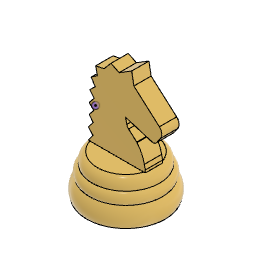
knight-piece (Autodesk Fusion 360 design; units mm, degrees)
Autodesk Fusion 360 part; units mm, degrees
sketch "Sketch1" plane through (0, 0, 0) normal (0, 1, 0) x (1, 0, 0)
  line L0 (0.63787, -5.613368) -> (1.322235, -4.705961)
  line L1 (1.781849, -13.501986) -> (2.054004, -12.134883)
  line L2 (4.431532, -15.195434) -> (3.230917, -13.790457)
  arc A0 (12.369222, -7.229903) -> (11.532634, -6.942255) centre (11.753991, -7.658845) ccw
  line L3 (0.654946, -7.413287) -> (1.44732, -6.605734)
  line L4 (7.495864, -6.835009) -> (8.909119, -5.586097)
  line L5 (11.532634, -6.942255) -> (6.964148, -8.353478)
  line L6 (12.782214, -7.990364) -> (12.77555, -7.981881)
  line L7 (0.992877, -11.410262) -> (1.682411, -10.30367)
  line L8 (12.846864, -9.85003) -> (8.411678, -13.769464)
  line L9 (2.054004, -12.134883) -> (0.992877, -11.410262)
  line L10 (8.94361, -5.555616) -> (9.013978, -5.467489)
  line L11 (0.773914, -9.412249) -> (1.492016, -8.460111)
  line L12 (13.044505, -8.198462) -> (12.369222, -7.229903)
  arc A1 (8.964814, -5.528278) -> (10.23694, -2.89688) centre (4.129914, -1.567691) ccw
  line L13 (5.849674, -14.499572) -> (4.431532, -15.195434)
  line L14 (1.322235, -4.705961) -> (0.495264, -3.671767)
  line L15 (1.304006, -2.784416) -> (0.492137, -1.671328)
  arc A2 (12.846864, -9.85003) -> (13.044505, -8.198462) centre (12.01912, -8.913365) ccw
  line L16 (3.230917, -13.790457) -> (1.781849, -13.501986)
  line L17 (6.964148, -8.353478) -> (7.181578, -7.368735)
  line L18 (10.404418, -1.671328) -> (10.404418, -2.127392)
  arc A3 (7.495864, -6.835009) -> (7.181578, -7.368735) centre (8.158059, -7.584341) ccw
  line L19 (1.492016, -8.460111) -> (0.654946, -7.413287)
  line L20 (8.411678, -13.769464) -> (8.035252, -15.843654)
  line L21 (0.495264, -3.671767) -> (1.304006, -2.784416)
  line L22 (1.44732, -6.605734) -> (0.63787, -5.613368)
  line L23 (8.035252, -15.843654) -> (5.849674, -14.499572)
  arc A4 (8.909119, -5.586097) -> (8.964814, -5.528278) centre (8.578022, -5.211431) ccw
  line L24 (10.23694, -2.89688) -> (10.404418, -2.127392)
  line L25 (1.682411, -10.30367) -> (0.773914, -9.412249)
  line L26 (0.492137, -1.671328) -> (10.404418, -1.671328)
  constraint perpendicular L1 L16
  constraint perpendicular L3 L25
  constraint parallel L0 L11
  constraint parallel L14 L19
  constraint parallel L4 L8
  constraint tangent A1 L24
  constraint tangent L10 A1
  constraint tangent L4 A3
  constraint tangent L17 A3
  constraint tangent L4 A4
  constraint tangent A1 A4
  constraint tangent L8 A2
  constraint tangent L12 A2
  constraint tangent A0 L5
  constraint tangent A0 L12
  constraint perpendicular L18 L26
extrude "Extrude3" add sketch "Sketch1" along normal blind 3 contours L0 L1 L2 A0 L3 L4 L5 L7 L8 L9 L10 L11 L12 A1 L13 L14 L15 A2 L16 L17 L18 A3 L19 L20 L21 L22 L23 A4 L24 L25 L26 picked at (9.407563, -10.657657)
sketch "Sketch4" plane through (0, 0, 0) normal (0, 1, 0) x (1, 0, 0)
sketch "Sketch5" plane through (0, 0, 0) normal (0, 1, 0) x (1, 0, 0)
scale "Scale1" factor 2.2 about (3.230917, 0, 13.790457) bodies 1
sketch "Sketch6" plane through (0, 0, 0) normal (0, -1, 0) x (1, 0, 0)
  arc A0 (24.820812, 1.488068) -> (24.386, 5.121516) centre (22.564965, 3.060854) ccw
  line L0 (24.386, 5.121516) -> (14.628591, 13.744271)
  line L1 (14.628591, 13.744271) -> (13.800454, 18.30749)
  line L2 (13.800454, 18.30749) -> (8.992182, 15.35051)
  line L3 (8.992182, 15.35051) -> (5.87227, 16.881406)
  line L4 (5.87227, 16.881406) -> (3.230917, 13.790457)
  line L5 (3.230917, 13.790457) -> (0.042969, 13.155821)
  line L6 (0.042969, 13.155821) -> (0.641708, 10.148194)
  line L7 (0.641708, 10.148194) -> (-1.692769, 8.554027)
  line L8 (-1.692769, 8.554027) -> (-0.175795, 6.119526)
  line L9 (-0.175795, 6.119526) -> (-2.174489, 4.158398)
  line L10 (-2.174489, 4.158398) -> (-0.594666, 2.063694)
  line L11 (-0.594666, 2.063694) -> (-2.43622, -0.239317)
  line L12 (-2.43622, -0.239317) -> (-0.692995, -2.015934)
  line L13 (-0.692995, -2.015934) -> (-2.473786, -4.199139)
  line L14 (-2.473786, -4.199139) -> (-0.968182, -6.195434)
  line L15 (-0.968182, -6.195434) -> (-2.787519, -8.47066)
  line L16 (-2.787519, -8.47066) -> (-1.008287, -10.422834)
  line L17 (-1.008287, -10.422834) -> (-2.794399, -12.871628)
  line L18 (-2.794399, -12.871628) -> (19.012619, -12.871628)
  line L19 (19.012619, -12.871628) -> (19.012619, -11.868286)
  line L20 (19.012619, -11.868286) -> (18.644167, -10.175413)
  arc A1 (18.644167, -10.175413) -> (15.845491, -4.386338) centre (5.208711, -13.099629) ccw
  arc A2 (15.845491, -4.386338) -> (15.722963, -4.259136) centre (14.994548, -5.083401) ccw
  line L21 (15.722963, -4.259136) -> (12.613801, -1.511528)
  arc A3 (11.922372, -0.337331) -> (12.613801, -1.511528) centre (14.070629, 0.137002) ccw
  line L22 (11.922372, -0.337331) -> (11.444026, 1.829102)
  line L23 (11.444026, 1.829102) -> (21.494694, -1.275588)
  arc A4 (21.494694, -1.275588) -> (23.335188, -0.642761) centre (21.98168, 0.30091) ccw
  line L24 (23.335188, -0.642761) -> (24.820812, 1.488068)
  arc A5 through (21, -17, -3.5) (20.820206, -14.544008, -3.5) (19.012619, -12.871628, -3.5)
  arc A6 through (22, -21, -3.5) (22.454283, -18.76143, -3.5) (21, -17, -3.5)
  arc A7 through (23.10911, -27.871628, -3.5) (23.693939, -24.251913, -3.5) (22, -21, -3.5)
  line L25 (23.10911, -27.871628, -3.5) -> (8.10911, -27.871628, -3.5)
  line L26 (8.10911, -12.871628, -3.5) -> (19.012619, -12.871628, -3.5)
  line L27 (8.10911, -27.871628, -3.5) -> (8.10911, -12.871628, -3.5)
  arc A8 through (19.090812, -16.404182, -3.5) (19.074831, -15.547783, -3.5) (18.549007, -14.871628, -3.5)
  arc A9 through (19.090812, -16.404182, -3.5) (19.170925, -17.809001, -3.5) (20.1564, -18.813378, -3.5)
  arc A10 through (20.402293, -19.796949, -3.5) (20.513998, -19.246501, -3.5) (20.1564, -18.813378, -3.5)
  arc A11 through (20.402293, -19.796949, -3.5) (20.006006, -21.154875, -3.5) (20.607217, -22.435325, -3.5)
  arc A12 through (21.705297, -25.871628, -3.5) (21.586877, -24.015871, -3.5) (20.607217, -22.435325, -3.5)
  line L28 (21.705297, -25.871628, -3.5) -> (10.10911, -25.871628, -3.5)
  line L29 (10.10911, -14.871628, -3.5) -> (18.549007, -14.871628, -3.5)
  line L30 (10.10911, -25.871628, -3.5) -> (10.10911, -14.871628, -3.5)
  point P0 (19.012619, -17.871628)
  point P1 (23.10911, -24.871628)
revolve "Revolve2" add sketch "Sketch6" angle 360 about axis through (8.10911, 3.5, -27.871628) along (0, 0, 1) contours A5 A6 A7 L25 L26 L27 in plane through (0, 3.5, 0) normal (0, -1, 0) picked at (13.775777, 3.5, -27.204962)
